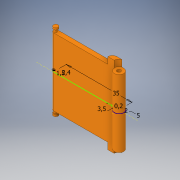
# Autodesk Inventor part: Bottom-Lip
Saved by Autodesk Inventor 2018.3 (Build 223284000, 284)
## iProperties
Created: 2018-05-20
Part Number: Bottom-Lip
Material: Generisch
Document SubType Name: Modeling
Designer: JochenAlt
Density: 1 g/cm^3
Appearance: Orange
Author: JochenAlt
Autodesk Inventor part; units mm, degrees
ref_plane "YZ Plane" through (0, 0, 0) normal (1, 0, 0) x (0, 1, 0)
ref_plane "XZ Plane" through (0, 0, 0) normal (0, 1, 0) x (-1, 0, 0)
ref_plane "XY Plane" through (0, 0, 0) normal (0, 0, 1) x (1, 0, 0)
sketch "Skizze1" plane through (0, 0, 0) normal (0, 0, 1) x (1, 0, 0)
  line L0 (0, 4.0964) -> (0, -3.5994) construction
  line L1 (-43.9572, 0) -> (10.2429, 0) construction
  circle A0 centre (0, 0) radius 2.5
  arc A1 (-34.9711, 2.5) -> (-35, 0.1003) centre (-35, 1.3003) ccw
  line L2 (-34.9711, 2.5) -> (0, 2.5)
  line L3 (-35, 0.1003) -> (-2.498, 0.1003)
  circle A2 centre (0, 0) radius 1
  arc A3 (-1.0198, 2.5) -> (-2.6981, 0.1003) centre (0, 0) ccw
  arc A4 (-3.5983, 2.5) -> (-5.998, 0.1003) centre (-3.5983, 0.1003) ccw
  circle A5 centre (-35, 1.3003) radius 0.75
  circle A6 centre (-35, 1.3003) radius 1.2
  dimension "d0" = 5
  dimension "d1" = 2.4
  dimension "d3" = 2
  dimension "d6" = 35
  dimension "d9" = 0.2
  dimension "d11" = 3.5
  dimension "d12" = 1.5
  constraints: 8 point on circle, 6 centre point, 5 coincident, 4 end point, 4 point on line, 3 tangent, 1 horizontal, 1 line through centre, 1 parallel, 3 other
  measures "d0" diameter of A0
  measures "d1" diameter of A1
  measures "d3" diameter of A2
  measures "d6" distance from line of L0 A1.centre
  measures "d9" radial gap between concentric circles of A0 A3
  measures "d11" distance of A4.end L3.end
  measures "d12" diameter of A5
extrude "Extrusion1" add sketch "Skizze1" along normal mid plane 36 contours A0 | A0 L3 A3 L2 | A3 L3 A4 L2 | A4 L3 A6 L2 | A6 A1 | A5
extrude "Extrusion2" add sketch "Skizze1" along normal mid plane 43 contours A3 L3 A4 L2
extrude "Extrusion3" add sketch "Skizze1" along normal mid plane 39 contours A5
extrude "Extrusion4" add sketch "Skizze1" along normal blind 1 from surface at 19.5 contours A6 A1 | A5
extrude "Extrusion5" add sketch "Skizze1" against normal blind 1 from surface at -19.5 contours A6 A1 | A5
